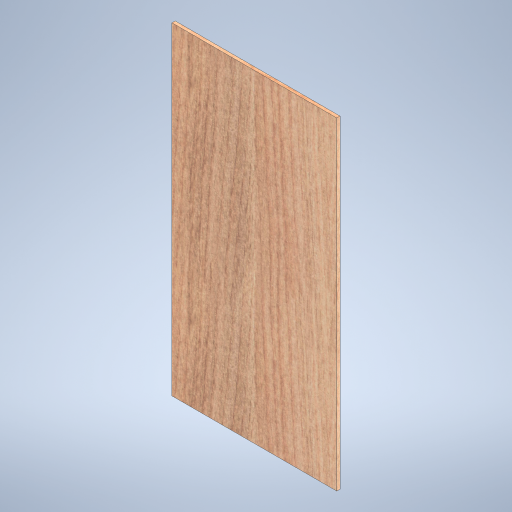
# Autodesk Inventor part: SIDE_PART_BOX
Saved by Autodesk Inventor 2023 (Build 270158000, 158)
## iProperties
Created: 2024-02-10
Part Number: SIDE_PART_BOX
Material: Wood (Birch)
Document SubType Name: Sheet Metal
Designer: vraco
Density: 0.55 g/cm^3
Sheet Metal Rule: Default_mm
Appearance: Birch - Natural Polished
Author: vraco
Autodesk Inventor part; units mm, degrees
ref_plane "YZ Plane" through (0, 0, 0) normal (1, 0, 0) x (0, 1, 0)
ref_plane "XZ Plane" through (0, 0, 0) normal (0, 1, 0) x (-1, 0, 0)
ref_plane "XY Plane" through (0, 0, 0) normal (0, 0, 1) x (1, 0, 0)
sketch "Sketch1" plane through (0, 0, 0) normal (0, 0, 1) x (1, 0, 0)
  line L0 (0, 480) -> (0, -80)
  line L1 (-40.8, 0) -> (244.8, 0)
  line L2 (0, 0) -> (204, 0)
  line L3 (204, 0) -> (204, 400)
  line L4 (204, 400) -> (0, 400)
  line L5 (0, 400) -> (0, 0)
  dimension "d0" = 204
  dimension "d1" = 400
  measures "d0" distance of L3.end L4.end
  measures "d1" distance of L2.end L3.end
extrude "Plate1" add sketch "Sketch1" along normal blind 4
equation "\"d2\" = Thickness"
equation "\"BendRadius\" = Thickness"
equation "\"BendReliefWidth\" = Thickness"
equation "\"BendReliefDepth\" = 0.5 * Thickness"
equation "\"CornerReliefSize\" = 4 * Thickness"
equation "\"MinimumRemnant\" = 2 * Thickness"
equation "\"TransitionRadius\" = BendRadius"
equation "\"JacobiRadiusSize\" = BendRadius"
equation "\"GapSize\" = Thickness"
equation "\"Thickness\" = 4"
body "Solid1"
